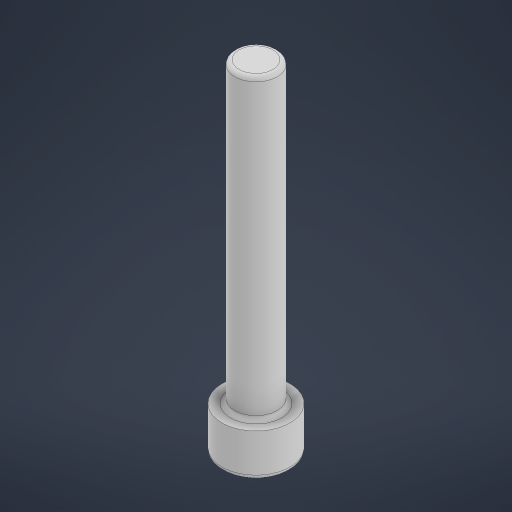
# Autodesk Inventor part: bulong5mm
Saved by Autodesk Inventor 2023 (Build 270158000, 158)
## iProperties
Created: 2023-09-13
Part Number: bulong5mm
Material: Generic
Document SubType Name: Modeling
Designer: philo
Density: 1 g/cm^3
Appearance: Default
Author: philo
Autodesk Inventor part; units mm, degrees
ref_plane "YZ Plane" through (0, 0, 0) normal (1, 0, 0) x (0, 1, 0)
ref_plane "XZ Plane" through (0, 0, 0) normal (0, 1, 0) x (-1, 0, 0)
ref_plane "XY Plane" through (0, 0, 0) normal (0, 0, 1) x (1, 0, 0)
sketch "Sketch1" plane through (0, 0, 0) normal (0, 1, 0) x (-1, 0, 0)
  circle A0 centre (0, 0) radius 4
  dimension "d0" = 8
  constraints: 1 centre point, 1 coincident
  measures "d0" diameter of A0
extrude "Extrusion1" add sketch "Sketch1" along normal blind 5
sketch "Sketch2" plane through (0, 5, 0) normal (0, 1, 0) x (1, 0, 0)
  circle A0 centre (0, 0) radius 2.5
  dimension "d3" = 5
  constraints: 1 centre point, 1 coincident
  measures "d3" diameter of A0
extrude "Extrusion2" add sketch "Sketch2" along normal blind 35
sketch "Sketch3" plane through (0, 0, 0) normal (0, -1, 0) x (1, 0, 0)
  line L0 (2.8865, -0.0416) -> (1.4072, -2.5205)
  line L1 (1.4072, -2.5205) -> (-1.4792, -2.479)
  line L2 (-1.4792, -2.479) -> (-2.8865, 0.0416)
  line L3 (-2.8865, 0.0416) -> (-1.4072, 2.5205)
  line L4 (-1.4072, 2.5205) -> (1.4792, 2.479)
  line L5 (1.4792, 2.479) -> (2.8865, -0.0416)
  point P0 (0, 0)
  point P1 (0, 0)
  dimension "d6" = 2.5
  constraints: 12 end point, 1 coincident, 13 other
  measures "d6" distance from line of L0 point (0, 0)
extrude "Extrusion3" cut sketch "Sketch3" against normal blind 3
fillet "Fillet1" radius 0.5 1 edges at (4, 0, 0)
fillet "Fillet2" radius 0.5 2 edges at (-2.5, 5, 0) (-2.5, 40, 0)
body "Solid1"
